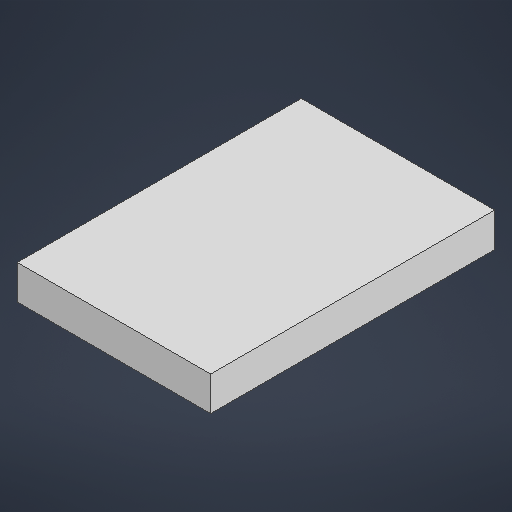
# Autodesk Inventor part: plocica
Saved by Autodesk Inventor 2025.2 (Build 292293000, 293)
## iProperties
Created: 2024-12-17
Part Number: plocica
Material: Generic
Document SubType Name: Modeling
Designer: antem
Density: 1 g/cm^3
Appearance: Default
Author: antem
Autodesk Inventor part; units mm, degrees
ref_plane "YZ Plane" through (0, 0, 0) normal (1, 0, 0) x (0, 1, 0)
ref_plane "XZ Plane" through (0, 0, 0) normal (0, 1, 0) x (-1, 0, 0)
ref_plane "XY Plane" through (0, 0, 0) normal (0, 0, 1) x (1, 0, 0)
sketch "Sketch1" plane through (0, 0, 0) normal (0, 0, 1) x (1, 0, 0)
  line L0 (-28.25, 41.5) -> (28.25, 41.5)
  line L1 (28.25, 41.5) -> (28.25, -41.5)
  line L2 (28.25, -41.5) -> (-28.25, -41.5)
  line L3 (-28.25, -41.5) -> (-28.25, 41.5)
  point P0 (0, 0)
  point P1 (28.25, 0)
  point P2 (0, 41.5)
  dimension "d0" = 83
  dimension "d1" = 56.5
  constraints: 8 end point, 2 midpoint, 2 parallel, 1 horizontal, 1 horizontal alignment, 1 perpendicular, 1 vertical alignment
  measures "d0" distance of L0.end L1.end
  measures "d1" distance of L0.start L0.end
extrude "Extrusion1" add sketch "Sketch1" along normal blind 10
body "Solid1"
